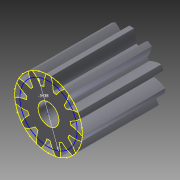
# Autodesk Inventor part: Spur Gear1
Saved by Autodesk Inventor 2012 (Build 160160000, 160)
## iProperties
Created: 2012-02-22
Part Number: Spur Gear1
Material: Steel
Document SubType Name: Modeling
Designer: admin
Categories: <?xml version="1.0" encoding="UTF-16"?> <MemberInstance><Categories><FamilyTemplate><FamilyTemplateParameter ValueType="xs:double" Id="1" ObjectReferenceKey="da_z" ObjectType="kUserParameterObject"/><FamilyTemplateParameter ValueType="xs:double" Id="2" ObjectReferenceKey="da_b" ObjectType="kUserParameterObject"/><FamilyTemplateParameter ValueType="xs:double" Id="3" ObjectReferenceKey="da_beta" ObjectType="kUserParameterObject"/><FamilyTemplateParameter ValueType="xs:double" Id="4" ObjectReferenceKey="da_da" ObjectType="kUserParameterObject"/><FamilyTemplateParameter ValueType="xs:double" Id="5" ObjectReferenceKey="da_aw" ObjectType="kUserParameterObject"/><FamilyTemplateParameter ValueType="xs:string" Id="6" ObjectReferenceKey="EAIAABAAAAC/AAAAAAAAAIAAAAAAAAAA" ObjectType="83910656" SubObjectId="SurfaceGeometry"/></FamilyTemplate><ParamToTemplateMap><ParamToTemplate CategoryParameter="//CategoryParameter[@InternalName='046C89C9-8512-4d59-83FE-43B91F4F132A']" TemplateParameter="1"/><ParamToTemplate CategoryParameter="//CategoryParameter[@InternalName='2552DF32-E462-4b46-AEBF-C6C7768E72AC']" TemplateParameter="2"/><ParamToTemplate CategoryParameter="//CategoryParameter[@InternalName='C9EE641D-15FC-4fae-A226-E94C4372FDD7']" TemplateParameter="3"/><ParamToTemplate><ParamToTemplate CategoryParameter="//CategoryParameter[@InternalName='00B6519A-459B-49c7-AD84-2E56D39A5744']" ConstantValue="0.000000"/></ParamToTemplate><ParamToTemplate><ParamToTemplate CategoryParameter="//CategoryParameter[@InternalName='04B31F0E-C7A6-4894-AA32-9629BEFACF47']" ConstantValue="1.000000"/></ParamToTemplate><ParamToTemplate><ParamToTemplate CategoryParameter="//CategoryParameter[@InternalName='43CBEC2E-7847-49e7-A936-2F7889FCB2D9']" ConstantValue="0.250000"/></ParamToTemplate><ParamToTemplate><ParamToTemplate CategoryParameter="//CategoryParameter[@InternalName='B1EFC894-105D-4ebd-86BF-FA20ED196853']" ConstantValue="0.350000"/></ParamToTemplate><ParamToTemplate><ParamToTemplate CategoryParameter="//CategoryParameter[@InternalName='51175063-3D10-4879-93E8-6246FE8B403D']" ConstantValue="2060110000.000000"/></ParamToTemplate><ParamToTemplate><ParamToTemplate CategoryParameter="//CategoryParameter[@InternalName='A3A52E27-4454-46a9-B0BD-C932399B70AF']" ConstantValue="0.300000"/></ParamToTemplate><ParamToTemplate><ParamToTemplate CategoryParameter="//CategoryParameter[@InternalName='91B76062-C214-41d9-B1B9-14D2AB99603D']" ConstantValue="0.079375"/></ParamToTemplate><ParamToTemplate><ParamToTemplate CategoryParameter="//CategoryParameter[@InternalName='374E806E-8B8A-4dda-A9AA-1039D6500AD2']" ConstantValue="12.598425"/></ParamToTemplate><ParamToTemplate><ParamToTemplate CategoryParameter="//CategoryParameter[@InternalName='2D373A89-B862-43d6-8D0B-0CBF12AB9F6C']" ConstantValue="0.349066"/></ParamToTemplate><ParamToTemplate CategoryParameter="//CategoryParameter[@InternalName='37777632-D6A2-4fac-9D53-DB8ACD95C989']" TemplateParameter="4"/><ParamToTemplate CategoryParameter="//CategoryParameter[@InternalName='FD1017F1-B727-4f7e-9707-0F86F1FF9423']" TemplateParameter="5"/><ParamToTemplate><ParamToTemplate CategoryParameter="//CategoryParameter[@InternalName='9E1B4470-B2D3-4ff1-B813-535BB4CDF51A']" ConstantValue="3520790.000000"/></ParamToTemplate><ParamToTemplate><ParamToTemplate CategoryParameter="//CategoryParameter[@InternalName='F8452263-BFF6-458c-9FB1-07C4B99E95CD']" ConstantValue="11389170.000000"/></ParamToTemplate><ParamToTemplate><ParamToTemplate CategoryParameter="//CategoryParameter[@InternalName='3E3BB259-FD49-497f-8171-6EBC954A3479']" ConstantValue="2.000000"/></ParamToTemplate><ParamToTemplate CategoryParameter="//CategoryParameter[@InternalName='27C3BAF2-7550-4e4b-AE2C-0DB134B7D9B7']" TemplateParameter="6"/></ParamToTemplateMap><Category DisplayName="Gear" InternalName="DC85795E-93AB-48d5-8EEE-5A27447B64BD" Mnemonic="Gear"><CategoryParameter DisplayName="z" InternalName="046C89C9-8512-4d59-83FE-43B91F4F132A" Mnemonic="z"/><CategoryParameter DisplayName="b" InternalName="2552DF32-E462-4b46-AEBF-C6C7768E72AC" Mnemonic="b"/><CategoryParameter DisplayName="||b|" InternalName="C9EE641D-15FC-4fae-A226-E94C4372FDD7" Mnemonic="beta"/><CategoryParameter DisplayName="x" InternalName="00B6519A-459B-49c7-AD84-2E56D39A5744" Mnemonic="x"/><CategoryParameter DisplayName="a*" InternalName="04B31F0E-C7A6-4894-AA32-9629BEFACF47" Mnemonic="a"/><CategoryParameter DisplayName="c*" InternalName="43CBEC2E-7847-49e7-A936-2F7889FCB2D9" Mnemonic="c"/><CategoryParameter DisplayName="r|.f|*" InternalName="B1EFC894-105D-4ebd-86BF-FA20ED196853" Mnemonic="rf"/><CategoryParameter DisplayName="E" InternalName="51175063-3D10-4879-93E8-6246FE8B403D" Mnemonic="E"/><CategoryParameter DisplayName="||m|" InternalName="A3A52E27-4454-46a9-B0BD-C932399B70AF" Mnemonic="mi"/><Category DisplayName="SpurGear" InternalName="26C5A22E-A91E-4dfd-A3B3-23CCAFAE1764" Mnemonic="SpurGear"><CategoryParameter DisplayName="m" InternalName="91B76062-C214-41d9-B1B9-14D2AB99603D" Mnemonic="m"/><CategoryParameter DisplayName="P" InternalName="374E806E-8B8A-4dda-A9AA-1039D6500AD2" Mnemonic="PP"/><CategoryParameter DisplayName="||a|" InternalName="2D373A89-B862-43d6-8D0B-0CBF12AB9F6C" Mnemonic="alpha"/><CategoryParameter DisplayName="d|.a|" InternalName="37777632-D6A2-4fac-9D53-DB8ACD95C989" Mnemonic="da"/><CategoryParameter DisplayName="a|.w|" InternalName="FD1017F1-B727-4f7e-9707-0F86F1FF9423" Mnemonic="aw"/><CategoryParameter DisplayName="||s||.Flim|" InternalName="9E1B4470-B2D3-4ff1-B813-535BB4CDF51A" Mnemonic="sFlim"/><CategoryParameter DisplayName="||s||.Hlim|" InternalName="F8452263-BFF6-458c-9FB1-07C4B99E95CD" Mnemonic="sHlim"/><CategoryParameter DisplayName="type" InternalName="3E3BB259-FD49-497f-8171-6EBC954A3479" Mnemonic="type"/><CategoryParameter DisplayName="PitchDiameter" InternalName="27C3BAF2-7550-4e4b-AE2C-0DB134B7D9B7" Mnemonic="IDS_PITCHDIAM"/></Category></Category></Categories></MemberInstance>
Density: 7.85 g/cm^3
Mass: 5.16007 g
Surface Area: 9.3079 cm^2
Volume: 0.657334 cm^3
CustomPartVersion: 1
Author: admin
Autodesk Inventor part; units mm, degrees
sketch "Sketch1" plane through (0, 0, 0) normal (0, 0, 1) x (1, 0, 0)
  circle A0 centre (0, 0) radius 5.1594
  dimension "d0" = 10.3187
  constraints: 1 centre point
  measures "d0" diameter of A0
extrude "Extrusion1" add sketch "Sketch1" along normal blind 12.7
sketch "Sketch2" plane through (0, 0, 0) normal (0, 0, -1) x (-1, 0, 0)
  circle A0 centre (0, 0) radius 5.1594 projected
  circle A1 centre (0, 0) radius 4.3656
  dimension "d3" = 8.7312
  constraints: 1 centre point, 1 coincident
  measures "d3" diameter of A1
surface extrude "Pitch Diameter" sketch "Sketch2" against normal through all shown no curves A1
ref_plane "Work Plane1" through (0, 0, 0) normal (1, 0, 0) x (0, 1, 0)
ref_plane "Work Plane2" through (0, 0, 0) normal (0.959493, 0.2817326, 0) x (0, 0, 1)
ref_plane "Work Plane3" through (0, 0, 6.35) normal (0, 0, -1) x (-1, 0, 0)
spur gear teeth "Spur Gear" teeth 11 pitch diameter 8.7313 tip diameter 10.3188 root diameter 6.7469 face width 12.7 start plane through (0, 0, 0) normal (0, 0, -1) x (-1, 0, 0)
sketch "Sketch3" plane through (0, 0, 12.7) normal (0, 0, 1) x (1, 0, 0)
  arc A0 (-3.0919, 4.1303) -> (-2.3854, 2.3854) centre (1.4657, 4.9602) ccw projected
  arc A1 (-2.3854, 2.3854) -> (-2.7006, 2.0216) centre (0, 0) ccw projected
  arc A2 (-2.7006, 2.0216) -> (-4.5283, 2.4726) centre (-4.7011, -2.1567) ccw projected
  circle A3 centre (0, 0) radius 5.1594 projected
  arc A4 (-4.8341, 1.803) -> (-3.2963, 0.7171) centre (-1.4487, 4.9652) ccw projected
  arc A5 (-3.2963, 0.7171) -> (-3.3648, 0.2407) centre (0, 0) ccw projected
  arc A6 (-3.3648, 0.2407) -> (-5.1462, -0.3681) centre (-2.7888, -4.3559) ccw projected
  circle A7 centre (0, 0) radius 5.1594 projected
  arc A8 (-5.0415, -1.0967) -> (-3.1607, -1.1789) centre (-3.9031, 3.3938) ccw projected
  arc A9 (-3.1607, -1.1789) -> (-2.9608, -1.6167) centre (0, 0) ccw projected
  arc A10 (-2.9608, -1.6167) -> (-4.1303, -3.0919) centre (0.0089, -5.1722) ccw projected
  circle A11 centre (0, 0) radius 5.1594 projected
  arc A12 (-3.6482, -3.6482) -> (-2.0216, -2.7006) centre (-5.1183, 0.7449) ccw projected
  arc A13 (-2.0216, -2.7006) -> (-1.6167, -2.9608) centre (0, 0) ccw projected
  arc A14 (-1.6167, -2.9608) -> (-1.803, -4.8341) centre (2.8037, -4.3463) ccw projected
  circle A15 centre (0, 0) radius 5.1594 projected
  arc A16 (-1.0967, -5.0415) -> (-0.2407, -3.3648) centre (-4.7085, -2.1405) ccw projected
  arc A17 (-0.2407, -3.3648) -> (0.2407, -3.3648) centre (0, 0) ccw projected
  arc A18 (0.2407, -3.3648) -> (1.0967, -5.0415) centre (4.7085, -2.1405) ccw projected
  circle A19 centre (0, 0) radius 5.1594 projected
  arc A20 (1.803, -4.8341) -> (1.6167, -2.9608) centre (-2.8037, -4.3463) ccw projected
  arc A21 (1.6167, -2.9608) -> (2.0216, -2.7006) centre (0, 0) ccw projected
  arc A22 (2.0216, -2.7006) -> (3.6482, -3.6482) centre (5.1183, 0.7449) ccw projected
  circle A23 centre (0, 0) radius 5.1594 projected
  arc A24 (4.1303, -3.0919) -> (2.9608, -1.6167) centre (-0.0089, -5.1722) ccw projected
  arc A25 (2.9608, -1.6167) -> (3.1607, -1.1789) centre (0, 0) ccw projected
  arc A26 (3.1607, -1.1789) -> (5.0415, -1.0967) centre (3.9031, 3.3938) ccw projected
  circle A27 centre (0, 0) radius 5.1594 projected
  arc A28 (5.1462, -0.3681) -> (3.3648, 0.2407) centre (2.7888, -4.3559) ccw projected
  arc A29 (3.3648, 0.2407) -> (3.2963, 0.7171) centre (0, 0) ccw projected
  arc A30 (3.2963, 0.7171) -> (4.8341, 1.803) centre (1.4487, 4.9652) ccw projected
  circle A31 centre (0, 0) radius 5.1594 projected
  arc A32 (4.5283, 2.4726) -> (2.7006, 2.0216) centre (4.7011, -2.1567) ccw projected
  arc A33 (2.7006, 2.0216) -> (2.3854, 2.3854) centre (0, 0) ccw projected
  arc A34 (2.3854, 2.3854) -> (3.0919, 4.1303) centre (-1.4657, 4.9602) ccw projected
  circle A35 centre (0, 0) radius 5.1594 projected
  arc A36 (2.4726, 4.5283) -> (1.1789, 3.1607) centre (5.1208, 0.7273) ccw projected
  arc A37 (1.1789, 3.1607) -> (0.7171, 3.2963) centre (0, 0) ccw projected
  arc A38 (0.7171, 3.2963) -> (0.3681, 5.1462) centre (-3.9147, 3.3804) ccw projected
  circle A39 centre (0, 0) radius 5.1594 projected
  arc A40 (-0.3681, 5.1462) -> (-0.7171, 3.2963) centre (3.9147, 3.3804) ccw projected
  arc A41 (-0.7171, 3.2963) -> (-1.1789, 3.1607) centre (0, 0) ccw projected
  arc A42 (-1.1789, 3.1607) -> (-2.4726, 4.5283) centre (-5.1208, 0.7273) ccw projected
  circle A43 centre (0, 0) radius 5.1594 projected
sketch "Sketch4" plane through (0, 0, 12.7) normal (0, 0, 1) x (1, 0, 0)
  arc A0 (-3.0919, 4.1303) -> (-2.3854, 2.3854) centre (1.4657, 4.9602) ccw projected
  arc A1 (-2.3854, 2.3854) -> (-2.7006, 2.0216) centre (0, 0) ccw projected
  arc A2 (-2.7006, 2.0216) -> (-4.5283, 2.4726) centre (-4.7011, -2.1567) ccw projected
  circle A3 centre (0, 0) radius 5.1594 projected
  arc A4 (-4.8341, 1.803) -> (-3.2963, 0.7171) centre (-1.4487, 4.9652) ccw projected
  arc A5 (-3.2963, 0.7171) -> (-3.3648, 0.2407) centre (0, 0) ccw projected
  arc A6 (-3.3648, 0.2407) -> (-5.1462, -0.3681) centre (-2.7888, -4.3559) ccw projected
  circle A7 centre (0, 0) radius 5.1594 projected
  arc A8 (-5.0415, -1.0967) -> (-3.1607, -1.1789) centre (-3.9031, 3.3938) ccw projected
  arc A9 (-3.1607, -1.1789) -> (-2.9608, -1.6167) centre (0, 0) ccw projected
  arc A10 (-2.9608, -1.6167) -> (-4.1303, -3.0919) centre (0.0089, -5.1722) ccw projected
  circle A11 centre (0, 0) radius 5.1594 projected
  arc A12 (-3.6482, -3.6482) -> (-2.0216, -2.7006) centre (-5.1183, 0.7449) ccw projected
  arc A13 (-2.0216, -2.7006) -> (-1.6167, -2.9608) centre (0, 0) ccw projected
  arc A14 (-1.6167, -2.9608) -> (-1.803, -4.8341) centre (2.8037, -4.3463) ccw projected
  circle A15 centre (0, 0) radius 5.1594 projected
  arc A16 (-1.0967, -5.0415) -> (-0.2407, -3.3648) centre (-4.7085, -2.1405) ccw projected
  arc A17 (-0.2407, -3.3648) -> (0.2407, -3.3648) centre (0, 0) ccw projected
  arc A18 (0.2407, -3.3648) -> (1.0967, -5.0415) centre (4.7085, -2.1405) ccw projected
  circle A19 centre (0, 0) radius 5.1594 projected
  arc A20 (1.803, -4.8341) -> (1.6167, -2.9608) centre (-2.8037, -4.3463) ccw projected
  arc A21 (1.6167, -2.9608) -> (2.0216, -2.7006) centre (0, 0) ccw projected
  arc A22 (2.0216, -2.7006) -> (3.6482, -3.6482) centre (5.1183, 0.7449) ccw projected
  circle A23 centre (0, 0) radius 5.1594 projected
  arc A24 (4.1303, -3.0919) -> (2.9608, -1.6167) centre (-0.0089, -5.1722) ccw projected
  arc A25 (2.9608, -1.6167) -> (3.1607, -1.1789) centre (0, 0) ccw projected
  arc A26 (3.1607, -1.1789) -> (5.0415, -1.0967) centre (3.9031, 3.3938) ccw projected
  circle A27 centre (0, 0) radius 5.1594 projected
  arc A28 (5.1462, -0.3681) -> (3.3648, 0.2407) centre (2.7888, -4.3559) ccw projected
  arc A29 (3.3648, 0.2407) -> (3.2963, 0.7171) centre (0, 0) ccw projected
  arc A30 (3.2963, 0.7171) -> (4.8341, 1.803) centre (1.4487, 4.9652) ccw projected
  circle A31 centre (0, 0) radius 5.1594 projected
  arc A32 (4.5283, 2.4726) -> (2.7006, 2.0216) centre (4.7011, -2.1567) ccw projected
  arc A33 (2.7006, 2.0216) -> (2.3854, 2.3854) centre (0, 0) ccw projected
  arc A34 (2.3854, 2.3854) -> (3.0919, 4.1303) centre (-1.4657, 4.9602) ccw projected
  circle A35 centre (0, 0) radius 5.1594 projected
  arc A36 (2.4726, 4.5283) -> (1.1789, 3.1607) centre (5.1208, 0.7273) ccw projected
  arc A37 (1.1789, 3.1607) -> (0.7171, 3.2963) centre (0, 0) ccw projected
  arc A38 (0.7171, 3.2963) -> (0.3681, 5.1462) centre (-3.9147, 3.3804) ccw projected
  circle A39 centre (0, 0) radius 5.1594 projected
  arc A40 (-0.3681, 5.1462) -> (-0.7171, 3.2963) centre (3.9147, 3.3804) ccw projected
  arc A41 (-0.7171, 3.2963) -> (-1.1789, 3.1607) centre (0, 0) ccw projected
  arc A42 (-1.1789, 3.1607) -> (-2.4726, 4.5283) centre (-5.1208, 0.7273) ccw projected
  circle A43 centre (0, 0) radius 5.1594 projected
sketch "Sketch5" plane through (0, 0, 12.7) normal (0, 0, 1) x (1, 0, 0)
  circle A0 centre (0, 0) radius 5.1594 projected
  circle A1 centre (0, 0) radius 1.5964
  dimension "d20" = 3.1928
  constraints: 1 centre point, 1 coincident
  measures "d20" diameter of A1
extrude "Extrusion2" cut sketch "Sketch5" against normal blind 12.7 contours A1
sketch "Sketch6" plane through (0, 0, 12.7) normal (0, 0, 1) x (1, 0, 0)
  circle A0 centre (0, 0) radius 1.5964 projected
  arc A1 (-3.0919, 4.1303) -> (-2.3854, 2.3854) centre (1.4657, 4.9602) ccw projected
  arc A2 (-2.3854, 2.3854) -> (-2.7006, 2.0216) centre (0, 0) ccw projected
  arc A3 (-2.7006, 2.0216) -> (-4.5283, 2.4726) centre (-4.7011, -2.1567) ccw projected
  arc A4 (-4.5283, 2.4726) -> (-4.8341, 1.803) centre (0, 0) ccw projected
  arc A5 (-4.8341, 1.803) -> (-3.2963, 0.7171) centre (-1.4487, 4.9652) ccw projected
  arc A6 (-3.2963, 0.7171) -> (-3.3648, 0.2407) centre (0, 0) ccw projected
  arc A7 (-3.3648, 0.2407) -> (-5.1462, -0.3681) centre (-2.7888, -4.3559) ccw projected
  arc A8 (-5.1462, -0.3681) -> (-5.0415, -1.0967) centre (0, 0) ccw projected
  arc A9 (-5.0415, -1.0967) -> (-3.1607, -1.1789) centre (-3.9031, 3.3938) ccw projected
  arc A10 (-3.1607, -1.1789) -> (-2.9608, -1.6167) centre (0, 0) ccw projected
  arc A11 (-2.9608, -1.6167) -> (-4.1303, -3.0919) centre (0.0089, -5.1722) ccw projected
  arc A12 (-4.1303, -3.0919) -> (-3.6482, -3.6482) centre (0, 0) ccw projected
  arc A13 (-3.6482, -3.6482) -> (-2.0216, -2.7006) centre (-5.1183, 0.7449) ccw projected
  arc A14 (-2.0216, -2.7006) -> (-1.6167, -2.9608) centre (0, 0) ccw projected
  arc A15 (-1.6167, -2.9608) -> (-1.803, -4.8341) centre (2.8037, -4.3463) ccw projected
  arc A16 (-1.803, -4.8341) -> (-1.0967, -5.0415) centre (0, 0) ccw projected
  arc A17 (-1.0967, -5.0415) -> (-0.2407, -3.3648) centre (-4.7085, -2.1405) ccw projected
  arc A18 (-0.2407, -3.3648) -> (0.2407, -3.3648) centre (0, 0) ccw projected
  arc A19 (0.2407, -3.3648) -> (1.0967, -5.0415) centre (4.7085, -2.1405) ccw projected
  arc A20 (1.0967, -5.0415) -> (1.803, -4.8341) centre (0, 0) ccw projected
  arc A21 (1.803, -4.8341) -> (1.6167, -2.9608) centre (-2.8037, -4.3463) ccw projected
  arc A22 (1.6167, -2.9608) -> (2.0216, -2.7006) centre (0, 0) ccw projected
  arc A23 (2.0216, -2.7006) -> (3.6482, -3.6482) centre (5.1183, 0.7449) ccw projected
  arc A24 (3.6482, -3.6482) -> (4.1303, -3.0919) centre (0, 0) ccw projected
  arc A25 (4.1303, -3.0919) -> (2.9608, -1.6167) centre (-0.0089, -5.1722) ccw projected
  arc A26 (2.9608, -1.6167) -> (3.1607, -1.1789) centre (0, 0) ccw projected
  arc A27 (3.1607, -1.1789) -> (5.0415, -1.0967) centre (3.9031, 3.3938) ccw projected
  arc A28 (5.0415, -1.0967) -> (5.1462, -0.3681) centre (0, 0) ccw projected
  arc A29 (5.1462, -0.3681) -> (3.3648, 0.2407) centre (2.7888, -4.3559) ccw projected
  arc A30 (3.3648, 0.2407) -> (3.2963, 0.7171) centre (0, 0) ccw projected
  arc A31 (3.2963, 0.7171) -> (4.8341, 1.803) centre (1.4487, 4.9652) ccw projected
  arc A32 (4.8341, 1.803) -> (4.5283, 2.4726) centre (0, 0) ccw projected
  arc A33 (4.5283, 2.4726) -> (2.7006, 2.0216) centre (4.7011, -2.1567) ccw projected
  arc A34 (2.7006, 2.0216) -> (2.3854, 2.3854) centre (0, 0) ccw projected
  arc A35 (2.3854, 2.3854) -> (3.0919, 4.1303) centre (-1.4657, 4.9602) ccw projected
  arc A36 (3.0919, 4.1303) -> (2.4726, 4.5283) centre (0, 0) ccw projected
  arc A37 (2.4726, 4.5283) -> (1.1789, 3.1607) centre (5.1208, 0.7273) ccw projected
  arc A38 (1.1789, 3.1607) -> (0.7171, 3.2963) centre (0, 0) ccw projected
  arc A39 (0.7171, 3.2963) -> (0.3681, 5.1462) centre (-3.9147, 3.3804) ccw projected
  arc A40 (0.3681, 5.1462) -> (-0.3681, 5.1462) centre (0, 0) ccw projected
  arc A41 (-0.3681, 5.1462) -> (-0.7171, 3.2963) centre (3.9147, 3.3804) ccw projected
  arc A42 (-0.7171, 3.2963) -> (-1.1789, 3.1607) centre (0, 0) ccw projected
  arc A43 (-1.1789, 3.1607) -> (-2.4726, 4.5283) centre (-5.1208, 0.7273) ccw projected
  arc A44 (-2.4726, 4.5283) -> (-3.0919, 4.1303) centre (0, 0) ccw projected
  circle A45 centre (0, 0) radius 4.3663
  dimension "d23" = 8.7325
  constraints: 1 centre point, 1 coincident
  measures "d23" diameter of A45
equation "\"d0\" = da_da"
equation "\"d3\" = da_dw"
equation "\"da_da\" = 10.31875"
equation "\"da_dw\" = 8.73125"
body "Solid1"
body "Srf1"
